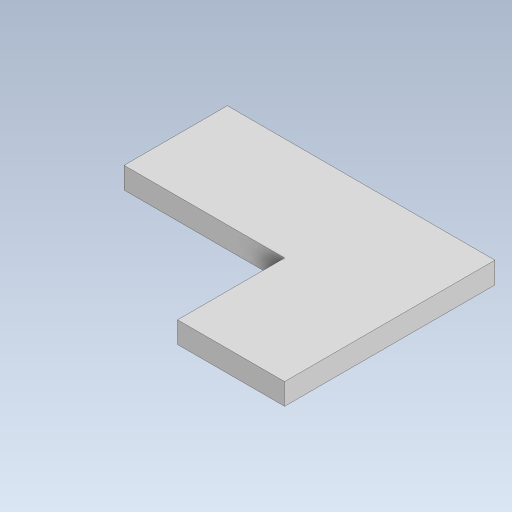
# Autodesk Inventor part: Bracket Motor Lifter
Saved by Autodesk Inventor 2023.5 (Build 275446000, 446)
## iProperties
Created: 2025-09-06
Part Number: Bracket Motor Lifter
Material: Generic
Document SubType Name: Modeling
Designer: Guntur
Density: 1 g/cm^3
Appearance: Default
Author: Guntur
## iProperties of the stored document Bracket Motor Lifter_3DPrint.ipt
Created: 2025-09-06
Part Number: Bracket Motor Lifter_3DPrint
Material: Generic
Document SubType Name: Modeling
Designer: Guntur
Density: 1 g/cm^3
Appearance: Default
Author: Guntur
Autodesk Inventor part; units mm, degrees
ref_plane "YZ Plane" through (0, 0, 0) normal (1, 0, 0) x (0, 1, 0)
ref_plane "XZ Plane" through (0, 0, 0) normal (0, 1, 0) x (-1, 0, 0)
ref_plane "XY Plane" through (0, 0, 0) normal (0, 0, 1) x (1, 0, 0)
sketch "Sketch1" plane through (0, 0, 0) normal (0, 1, 0) x (-1, 0, 0)
  line L0 (25, 19.65) -> (-25, 19.65)
  line L1 (-25, 19.65) -> (-25, -19.65)
  line L2 (-25, -19.65) -> (25, -19.65)
  line L3 (25, -19.65) -> (25, 19.65)
  line L4 (25, 19.65) -> (-25, -19.65) construction
  line L5 (-25, 19.65) -> (25, -19.65) construction
  line L6 (25, 19.65) -> (-5, 19.65)
  line L7 (-5, 19.65) -> (-5, -0.35)
  line L8 (-5, -0.35) -> (25, -0.35)
  line L9 (25, -0.35) -> (25, 19.65)
  point P0 (0, 0)
  dimension "d0" = 50
  dimension "d1" = 39.3
  dimension "d2" = 30
  dimension "d3" = 20
  constraints: 20 end point, 4 parallel, 2 horizontal, 2 midpoint, 2 perpendicular
  measures "d0" distance of L2.end L1.end
  measures "d1" distance of L1.end L0.end
  measures "d2" distance of L8.end L7.end
  measures "d3" distance of L7.end L6.end
extrude "Extrusion1" add sketch "Sketch1" along normal blind 4 contours L7 L8 L3 L2 L1 L0
body "Solid1"
